drawer_pin (Autodesk Fusion 360 design; units mm, degrees)
Autodesk Fusion 360 part; units mm, degrees
note: some values were not read from the file. Set by a fixed rule: which sketch regions a step uses.
sketch "Sketch1" plane through (0, 0, 0) normal (0, 1, 0) x (1, 0, 0)
  circle A0 centre (0, 0) radius 6
  circle A1 centre (0, 0) radius 2.9
  circle A2 centre (-30, 0) radius 6
  circle A3 centre (-30, 0) radius 2.9
  line L0 (0, 0) -> (-30, 0)
  line L1 (-31.2, 2.6401) -> (-31.2, -2.6401)
  dimension "d1" = 12
  dimension "d2" = 5.8
  dimension "d9" = 30
  dimension "d10" = 12
  dimension "d11" = 5.8
  dimension "d12" = 1.2
  constraint coincident A0.centre A1.centre
  constraint concentric A0 A1
  constraint concentric A2 A3
  constraint horizontal L0
  constraint coincident A2.centre A3.centre
  constraint coincident A3 L1.start
  constraint coincident A3 L1.end
  constraint vertical L1
  measures "d1" diameter of A0
  measures "d2" diameter of A1
  measures "d9" distance of A0.centre A2.centre
  measures "d10" diameter of A2
  measures "d11" diameter of A3
  measures "d12" distance of A2.centre L1
extrude "Extrude1" add sketch "Sketch1" along normal blind 4 contours A0 | A1 | A2 | A3 L1 | A3 L1 makes body 1 at (5.9925, 1.3333, 0.2991) makes body 2 at (-24.0075, 2.6667, 0.2991)
extrude "Extrude2" add sketch "Sketch1" against normal blind 10 contours A1 | A3 L1 picked at (-29.8333, 0) bodies 1 2
chamfer "Chamfer1" distance 3 angle 45 2 edges at (-5.594, 4, 2.1697) (-35.594, 4, 2.1697) on bodies 1 2
chamfer "Chamfer2" distance 1 angle 45 3 edges at (-2.7037, -10, -1.0487) (-27.1, -10, 0) (-31.2, -10, 0) on bodies 1 2
equation "d10 = d1"
equation "d11 = d2"
